Autodesk Fusion 360 part; units mm, degrees
(part 2 of 2)
  arc A348 (19.6906, 54.0234) -> (20.5376, 54.2169) centre (19.9646, 54.7751) ccw
  arc A349 (23.5573, 57.3171) -> (20.5376, 54.2169) centre (35.8584, 42.315) ccw
  arc A350 (23.6197, 57.3246) -> (23.5573, 57.3171) centre (23.5931, 57.2822) ccw
  line L119 (23.6113, 57.3288) -> (24.165, 57.0977)
  arc A351 (24.1947, 57.051) -> (24.1561, 57.1006) centre (24.1447, 57.052) ccw
  arc A352 (24.1348, 52.894) -> (24.5721, 51.9852) centre (24.9131, 52.7089) ccw
  arc A353 (18.47, 54.9556) -> (18.0987, 59.2675) centre (-0.9241, 55.4575) ccw
  arc A354 (13.9357, 55.7857) -> (14.7579, 56.0666) centre (14.1296, 56.5619) ccw
  arc A355 (17.437, 59.4656) -> (14.7579, 56.0666) centre (31.2389, 45.8314) ccw
  arc A356 (17.4983, 59.4795) -> (17.437, 59.4656) centre (17.4763, 59.4346) ccw
  line L120 (17.4895, 59.4828) -> (18.0643, 59.3108)
  arc A357 (18.0987, 59.2675) -> (18.0551, 59.3128) centre (18.0488, 59.2632) ccw
  arc A358 (18.4737, 55.127) -> (19.0036, 54.2689) centre (19.267, 55.0243) ccw
  arc A359 (12.6244, 56.5852) -> (11.8044, 60.8347) centre (-6.7159, 55.0571) ccw
  arc A360 (8.0282, 56.9368) -> (8.8165, 57.3021) centre (8.1399, 57.729) ccw
  arc A361 (11.1256, 60.9625) -> (8.8165, 57.3021) centre (26.277, 48.8457) ccw
  arc A362 (11.1851, 60.9827) -> (11.1256, 60.9625) centre (11.1679, 60.9358) ccw
  line L121 (11.176, 60.9851) -> (11.7657, 60.8741)
  arc A363 (11.8044, 60.8347) -> (11.7563, 60.8752) centre (11.7553, 60.8252) ccw
  arc A364 (12.6101, 56.7561) -> (13.2268, 55.958) centre (13.4099, 56.7368) ccw
  arc A365 (6.6404, 57.5949) -> (5.3807, 61.7353) centre (-12.4341, 54.0535) ccw
  arc A366 (2.0327, 57.4641) -> (2.7785, 57.9098) centre (2.061, 58.2636) ccw
  arc A367 (4.6924, 61.7914) -> (2.7785, 57.9098) centre (21.0273, 51.3248) ccw
  arc A368 (4.7494, 61.8178) -> (4.6924, 61.7914) centre (4.7372, 61.7693) ccw
  line L122 (4.7401, 61.8193) -> (5.3381, 61.7705)
  arc A369 (5.3807, 61.7353) -> (5.3287, 61.7706) centre (5.3329, 61.7208) ccw
  arc A370 (6.6084, 57.7633) -> (7.3051, 57.0341) centre (7.4058, 57.8277) ccw
  point P0 (0.8876, 57.816)
  point P1 (-3.5861, 57.7115)
  dimension "d1" = 4.5
  dimension "d2" = 102
  dimension "d3" = 110
  dimension "d4" = 11.77
  dimension "d6" = 360
  dimension "d7" = 124
  dimension "d8" = 115
  dimension "d9" = 16.625
  dimension "d10" = 25.25
  dimension "d12" = 360
  dimension "d13" = 0.6
  dimension "d14" = 0.1
  dimension "d16" = 5.4
  dimension "d17" = 1.6
  dimension "d19" = 360
  constraint coincident A0.centre A1.centre
  constraint concentric A0 A1
  constraint coincident A1 L0.start
  constraint coincident A2 L0.end
  constraint vertical L0
  constraint coincident A1 L1.end
  constraint concentric A0 A3
  constraint concentric A2 A4
  constraint vertical L60
  constraint coincident L60.end A5.centre
  constraint tangent L61 A15
  constraint vertical L61.end A15.centre
  constraint midpoint L61 L63.start
  constraint symmetric L62.start L62.end L63
  constraint coincident A4 L62.end
  constraint tangent A4 A12
  constraint symmetric L63 A15 A16
  constraint symmetric L63 A12 A14
  constraint symmetric L61.start L61.end L63
  constraint symmetric L63 P0 P1
  constraint vertical L62.start A12.centre
  constraint coincident A3 L63.start
  constraint coincident A4 A12.start
  constraint symmetric L63 A11.end A13.start
  constraint symmetric L63 A11.start A13.end
  constraint symmetric L63 A11 A13
  constraint coincident A4 A14.end
  constraint coincident A13 A14.start
  constraint coincident A3 A15.end
  constraint coincident A3 A16.start
  measures "d1" diameter of A0
  measures "d2" diameter of A1
  measures "d3" diameter of A2
  measures "d4" distance of L0.end L1.end
  measures "d7" diameter of A3
  measures "d8" diameter of A4
  measures "d9" distance of L2.end L60.end
  measures "d10" diameter of A5
  measures "d13" distance of L61.start L61.end
  measures "d14" diameter of A15
  measures "d16" distance of L62.start L62.end
  measures "d17" diameter of A12
extrude "Extrude1" add sketch "bottom" along normal blind 5 contours A1 L0 L1 makes body 1
extrude "Extrude2" add sketch "bottom" along normal blind 5 contours A1 bodies 1
pattern_circular "C-Pattern1" count 30 over 360 about axis through (0, 0, 0) along (0, 0, 1) of "Extrude1"
extrude "Extrude3" add sketch "bottom" along normal blind 13 contours A1 A2 L0 L2 bodies 1
pattern_circular "C-Pattern2" count 30 over 360 about axis through (0, 0, 0) along (0, 0, 1) of "Extrude3"
extrude "Extrude4" add sketch "bottom" along normal blind 13 separate body contours A3 A4 L61 A11 A12 A13 A14 A15 A16 makes body 2
pattern_circular "C-Pattern3" count 60 over 360 about axis through (0, 0, 0) along (0, 0, 1) of "Extrude4" makes body 3 at (-5.2983, 57.2554, 4.3333) makes body 4 at (-11.2541, 56.3879, 4.3333) makes body 5 at (-17.0866, 54.9026, 4.3333) makes body 6 at (-22.7318, 52.8158, 4.3333) makes body 7 at (-28.1281, 50.1504, 4.3333) makes body 8 at (-33.2161, 46.9355, 4.3333) makes body 9 at (-37.9403, 43.2063, 4.3333) makes body 10 at (-42.2487, 39.0038, 8.6667) makes body 11 at (-46.0943, 34.3739, 4.3333) makes body 12 at (-49.4348, 29.3675, 4.3333) makes body 13 at (-52.2338, 24.0392, 8.6667) makes body 14 at (-54.4604, 18.4476, 4.3333) makes body 15 at (-56.0904, 12.6539, 4.3333) makes body 16 at (-57.1058, 6.7216, 4.3333) makes body 17 at (-57.4955, 0.7156, 4.3333) makes body 18 at (-57.2554, -5.2983, 4.3333) makes body 19 at (-56.3879, -11.2541, 4.3333) makes body 20 at (-54.9026, -17.0866, 4.3333) makes body 21 at (-52.8158, -22.7318, 4.3333) makes body 22 at (-50.1504, -28.1281, 4.3333) makes body 23 at (-46.9355, -33.2161, 4.3333) makes body 24 at (-43.2063, -37.9403, 4.3333) makes body 25 at (-39.0038, -42.2487, 8.6667) makes body 26 at (-34.3739, -46.0943, 4.3333) makes body 27 at (-29.3675, -49.4348, 4.3333) makes body 28 at (-24.0392, -52.2338, 8.6667) makes body 29 at (-18.4476, -54.4604, 4.3333) makes body 30 at (-12.6539, -56.0904, 4.3333) makes body 31 at (-6.7216, -57.1058, 4.3333) makes body 32 at (-0.7156, -57.4955, 4.3333) makes body 33 at (5.2983, -57.2554, 4.3333) makes body 34 at (11.2541, -56.3879, 4.3333) makes body 35 at (17.0866, -54.9026, 4.3333) makes body 36 at (22.7318, -52.8158, 4.3333) makes body 37 at (28.1281, -50.1504, 4.3333) makes body 38 at (33.2161, -46.9355, 4.3333) makes body 39 at (37.9403, -43.2063, 4.3333) makes body 40 at (42.2487, -39.0038, 4.3333) makes body 41 at (46.0943, -34.3739, 4.3333) makes body 42 at (49.4348, -29.3675, 4.3333) makes body 43 at (52.2338, -24.0392, 8.6667) makes body 44 at (54.4604, -18.4476, 4.3333) makes body 45 at (56.0904, -12.6539, 4.3333) makes body 46 at (57.1058, -6.7216, 4.3333) makes body 47 at (57.4955, -0.7156, 4.3333) makes body 48 at (57.2554, 5.2983, 4.3333) makes body 49 at (56.3879, 11.2541, 4.3333) makes body 50 at (54.9026, 17.0866, 4.3333) makes body 51 at (52.8158, 22.7318, 4.3333) makes body 52 at (50.1504, 28.1281, 4.3333) makes body 53 at (46.9355, 33.2161, 4.3333) makes body 54 at (43.2063, 37.9403, 4.3333) makes body 55 at (39.0038, 42.2487, 8.6667) makes body 56 at (34.3739, 46.0943, 4.3333) makes body 57 at (29.3675, 49.4348, 4.3333) makes body 58 at (24.0392, 52.2338, 8.6667) makes body 59 at (18.4476, 54.4604, 4.3333) makes body 60 at (12.6539, 56.0904, 4.3333) makes body 61 at (6.7216, 57.1058, 4.3333)
extrude "Extrude5" add sketch "bottom" along normal blind 13 contours A4 bodies 1 2 3 4 5 6 7 8 9 10 11 12 13 14 15 16 17 18 19 20 21 22 23 24 25 26 27 28 29 30 31 32 33 34 35 36 37 38 39 40 41 42 43 44 45 46 47 48 49 50 51 52 53 54 55 56 57 58 59 60 61
fillet "Fillet1" radius 1 2 edges at (17.9977, 21.7551, 5) (17.9977, 21.7551, 0) on bodies 1
fillet "Fillet2" radius 1 5 edges at (-41.539, -12.6243, 5) (-11.7681, -29.8096, 5) (-41.5415, 21.7507, 5) (-11.7732, 38.9404, 5) (18.0003, -12.6199, 5) on bodies 1
fillet "Fillet3" radius 1 5 edges at (18.0003, -12.6199, 0) (-11.7681, -29.8096, 0) (-41.539, -12.6243, 0) (-41.5415, 21.7507, 0) (-11.7732, 38.9404, 0) on bodies 1
equation "d9 = ( ( 25.25 / 2 ) * 1 mm ) + 4 mm"
named bodies: "SpringBarrel"

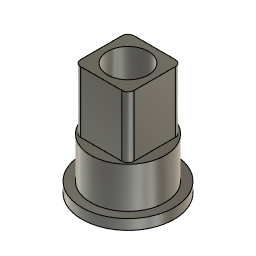
design "WindingSteam"
Autodesk Fusion 360 part; units mm, degrees
sketch "bottom" plane through (0, 0, 0) normal (0, 0, 1) x (1, 0, 0)
  circle A0 centre (0, 0) radius 2.25
  circle A1 centre (0, 0) radius 5
  line L0 (5.04, 6.54) -> (-5.04, 6.54)
  line L1 (-6.54, 5.04) -> (-6.54, -5.04)
  line L2 (-5.04, -6.54) -> (5.04, -6.54)
  line L3 (6.54, -5.04) -> (6.54, 5.04)
  line L4 (6.54, 6.54) -> (-6.54, -6.54) construction
  line L5 (-6.54, 6.54) -> (6.54, -6.54) construction
  arc A2 (-5.04, 6.54) -> (-6.54, 5.04) centre (-5.04, 5.04) ccw
  arc A3 (6.54, 5.04) -> (5.04, 6.54) centre (5.04, 5.04) ccw
  arc A4 (5.04, -6.54) -> (6.54, -5.04) centre (5.04, -5.04) ccw
  arc A5 (-6.54, -5.04) -> (-5.04, -6.54) centre (-5.04, -5.04) ccw
  circle A6 centre (0, 0) radius 9.1
  circle A7 centre (0, 0) radius 11.25
  dimension "d1" = 4.5
  dimension "d2" = 10
  dimension "d3" = 13.08
  dimension "d4" = 13.08
  dimension "d5" = 1.5
  dimension "d6" = 18.2
  dimension "d7" = 22.5
  constraint coincident A0.centre A1.centre
  constraint concentric A0 A1
  constraint horizontal L0
  constraint perpendicular L0 L1
  constraint parallel L0 L2
  constraint parallel L1 L3
  constraint coincident L4 A0.centre
  constraint coincident L5 A0.centre
  constraint coincident L5.start L0
  constraint coincident L5.start L1
  constraint tangent L0 A2
  constraint tangent L1 A2
  constraint coincident L4.start L0
  constraint coincident L4.start L3
  constraint tangent L0 A3
  constraint tangent L3 A3
  constraint equal A2 A3
  constraint coincident L5.end L3
  constraint coincident L5.end L2
  constraint tangent L3 A4
  constraint tangent L2 A4
  constraint equal A2 A4
  constraint coincident L4.end L2
  constraint coincident L4.end L1
  constraint tangent L2 A5
  constraint tangent L1 A5
  constraint equal A2 A5
  constraint concentric A1 A6
  constraint concentric A6 A7
  measures "d1" diameter of A0
  measures "d2" diameter of A1
  measures "d3" distance of L4.end L5.end
  measures "d4" distance of L5.start L4.end
  measures "d5" radius of A2
  measures "d6" diameter of A6
  measures "d7" diameter of A7
extrude "Extrude1" add sketch "bottom" along normal blind 27.5 and the other way blind -7.5 contours L0 L1 L2 L3 A2 A3 A4 A5
extrude "Extrude2" add sketch "bottom" along normal blind 12.5 and the other way blind -7.5 contours A1
extrude "Extrude3" add sketch "bottom" along normal blind 12.5 contours A6
extrude "Extrude4" add sketch "bottom" along normal blind 2.5 contours A7
equation "d12 = 5.00 mm + 7.50 mm"
named bodies: "WindingSteam"
